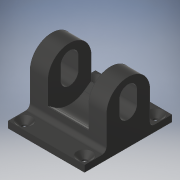
# Autodesk Inventor part: BT101_trajan20_21
Saved by Autodesk Inventor 2022.2 (Build 262287000, 287)
## iProperties
Company: HTBLA Kaindorf
RuleStatus: InUse
Created: 2022-08-03
Part Number: BT101_trajan20_21
Project: Zeichenmaschine_v2
Material: Kunststoff, undurchsichtig Schwarz
Description: halterung
Document SubType Name: Modeling
Designer: trajan20
Density: 0.952 g/cm^3
Appearance: Glatt - Schwarz
Mass: 10.1485 g
Surface Area: 60.7979 cm^2
Volume: 10.6602 cm^3
AfterDocNew0: iProperties-Editor_aufrufen
Author: jan
Keywords: 2021
Autodesk Inventor part; units mm, degrees
ref_plane "YZ Plane" through (0, 0, 0) normal (1, 0, 0) x (0, 1, 0)
ref_plane "XZ Plane" through (0, 0, 0) normal (0, 1, 0) x (-1, 0, 0)
ref_plane "XY Plane" through (0, 0, 0) normal (0, 0, 1) x (1, 0, 0)
sketch "Skizze3" plane through (0, 0, 0) normal (0, 0, 1) x (1, 0, 0)
  line L0 (0, 0) -> (-40, 0)
  line L1 (-40, 0) -> (-40, 35)
  line L2 (-40, 35) -> (0, 35)
  line L3 (0, 35) -> (0, 0)
  point P0 (-3.7, 3.7)
  dimension "d4" = 35
  dimension "d5" = 40
  dimension "d6" = 3.7
  dimension "d7" = 3.7
  constraints: 8 end point, 2 parallel, 1 horizontal, 1 perpendicular
  measures "d4" distance between parallel lines of L2 L0
  measures "d5" distance between parallel lines of L1 L3
  measures "d6" distance from line of L3 point (-3.7, 3.7)
  measures "d7" distance from line of L0 point (-3.7, 3.7)
sketch "Skizze4" plane through (0, 0, 0) normal (0, 1, 0) x (-1, 0, 0)
  line L0 (0, 0) -> (40, 0) projected
  line L1 (20, 0) -> (20, 25)
  line L2 (20, 18) -> (20, 12) construction
  line L3 (24, 18) -> (24, 12)
  line L4 (16, 12) -> (16, 18)
  arc A0 (24, 18) -> (16, 18) centre (20, 18) ccw
  arc A1 (16, 12) -> (24, 12) centre (20, 12) ccw
  circle A2 centre (20, 15) radius 10
  line L5 (30, 15) -> (30, 0)
  line L6 (10, 15) -> (10, 0)
  dimension "d9" = 10
  dimension "d10" = 8
  dimension "d11" = 6
  dimension "d12" = 10
  dimension "d13" = 10
  dimension "d46" = 12
  constraints: 14 end point, 7 point on circle, 6 tangent, 4 point on line, 3 centre point, 2 midpoint, 1 coincident, 1 parallel, 1 vertical
  measures "d9" distance of L1.end point (20, 15)
  measures "d10" distance between parallel lines of L4 L3
  measures "d11" distance of L2.start L2.end
  measures "d12" distance of L1.start L6.end
  measures "d13" distance of L1.start L5.end
  measures "d46" distance from line of L0 L2.end
extrude "Extrusion3" add sketch "Skizze4" along normal blind 35 contours L6 A2 L1 L0 | L1 A2 L5 L0 | A2 L1 A0 L4 A1 | L1 A1 L3 A0 A2
extrude "Extrusion4" add sketch "Skizze3" against normal blind 3
hole "Bohrung1" at (-3.7, 3.7, 0) direction (0, 0, -1) diameter 2.459 depth 8.8 countersink diameter 7 countersink angle 90
sketch "Skizze5" plane through (0, 0, 0) normal (1, 0, 0) x (0, 0, -1)
  line L0 (-25, 0) -> (-25, 35) projected
  line L1 (-25, 8.1) -> (0, 8.1)
  line L2 (0, 8.1) -> (0, 26.9)
  line L3 (0, 26.9) -> (-25, 26.9)
  line L4 (-25, 26.9) -> (-25, 8.1)
  line L5 (0, 0) -> (0, 35) projected
  point P0 (-25, 17.5)
  point P1 (-25, 26.9)
  point P2 (0, 17.5)
  point P3 (0, 17.5)
  dimension "d25" = 18.8
  constraints: 8 end point, 6 midpoint, 2 parallel, 1 horizontal, 1 perpendicular, 1 point on line
  measures "d25" distance between parallel lines of L3 L1
extrude "Extrusion5" cut sketch "Skizze5" against normal through all
pattern_linear "Rechteckige Anordnung1" count 2 spacing 32.6 along (-1, 0, 0) count 2 spacing 27.6 along (0, 1, 0) of "Bohrung1"
sketch "Skizze6" plane through (-20, 26.9, 15) normal (0, -1, 0) x (1, 0, 0)
  line L0 (-10, -15) -> (-10, 0) projected
  line L1 (10, 0) -> (10, -15) projected
  line L2 (10, -15) -> (-10, -15) projected
  arc A0 (-4, -3) -> (4, -3) centre (0, -3) ccw projected
  arc A1 (10, 0) -> (-10, 0) centre (0, 0) ccw projected
  line L3 (10, 0) -> (10, -15) projected
  line L4 (-10, -15) -> (-10, 0) projected
  circle A2 centre (0, -3) radius 11.5
  line L5 (-6.6647, -12.3719) -> (-10, -10)
  line L6 (10, 0) -> (10, -15) projected
  line L7 (10, -10) -> (6.6647, -12.3719)
  point P0 (20, -15)
  point P1 (-10, -10)
  dimension "d47" = 23
  dimension "d48" = 5
  dimension "d49" = 5
  constraints: 4 end point, 2 point on circle, 2 point on line, 2 tangent, 1 centre point, 1 coincident
  measures "d47" diameter of A2
  measures "d48" distance from line of L5.end L2
  measures "d49" distance from line of L7.start L2
extrude "Extrusion6" add sketch "Skizze6" along normal up to surface (18.8 mm away) contours L0 L5 A2 L7 L1 L2
fillet "Rundung4" radius 2 2 edges at (-10, 17.5, 0) (-30, 17.5, 0)
fillet "Rundung5" radius 0.2 2 edges at (-30, 17.5, 5) (-10, 17.5, 5)
equation "\"d7\" = d6"
equation "\"d13\" = d12"
equation "\"d14\" = d4"
equation "\"d31\" = d5 - 2 * d6"
equation "\"d34\" = d4 - 2 * d7"
